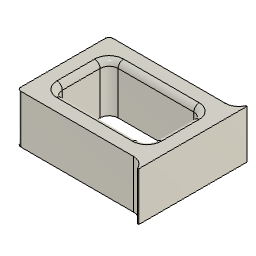
V0.2 Formbot Umbilical Panel Thermistor & 4-way Fan Bus v7 (Autodesk Fusion 360 design; units mm, degrees)
Autodesk Fusion 360 part; units mm, degrees
sketch "Fan Connector box" plane through (0, 0, 0) normal (0, 0, 1) x (1, 0, 0)
  line L0 (0, 0) -> (28.97, 0)
  line L1 (28.97, 0) -> (28.97, 7.7)
  line L2 (28.97, 7.7) -> (0, 7.7)
  line L3 (0, 7.7) -> (0, 0)
  dimension "d1" = 28.97
  dimension "d2" = 7.7
  constraint horizontal L0
  constraint vertical L1
  constraint horizontal L2
  constraint vertical L3
  constraint coincident L0.start L3.end
  measures "d1" distance of L0.start L0.end
  measures "d2" distance of L0.start L2.end
extrude "Extrude1" add sketch "Fan Connector box" along normal blind 6.5 makes body 1
shell "Shell1" thickness 1.2 outward yes removed faces 1 at (9.6567, 5.1333, 6.5) on bodies 1
chamfer "Chamfer1" distance 0.4 angle 45 4 edges at (14.485, 7.7, 6.5) (0, 3.85, 6.5) (14.485, 0, 6.5) (28.97, 3.85, 6.5) on bodies 1
sketch "v0.2 Formnot Umbilical Thermister Shroud" plane through (0, 0, 0) normal (0, 0, 1) x (1, 0, 0)
  line L0 (0, 23) -> (14.4, 23)
  line L1 (14.4, 23) -> (14.4, 12.8)
  line L2 (14.4, 12.8) -> (0, 12.8)
  line L3 (0, 12.8) -> (0, 23)
  circle A0 centre (12.9, 24.5) radius 1.5
  circle A1 centre (12.9, 11.3) radius 1.5
  line L4 (14.4, 12.8) -> (14.4, 11.3)
  line L5 (14.4, 23) -> (14.4, 24.5)
  dimension "d15" = 14.4
  dimension "d16" = 10.2
  dimension "d17" = 3
  dimension "d18" = 3
  constraint horizontal L0
  constraint vertical L1
  constraint horizontal L2
  constraint vertical L3
  constraint tangent L0 A0
  constraint tangent L1 A0
  constraint tangent L2 A1
  constraint tangent L1 A1
  constraint coincident A1 L4.end
  constraint tangent A1 L4
  constraint coincident A0 L5.end
  constraint tangent A0 L5
  measures "d15" distance of L0.start L0.end
  measures "d16" distance of L0.start L2.end
  measures "d17" diameter of A0
  measures "d18" diameter of A1
extrude "Extrude3" add sketch "v0.2 Formnot Umbilical Thermister Shroud" along normal blind 5.36 separate body contours L0 L1 L2 L3 | L0 A0 L5 | L2 A1 L4 makes body 2
shell "Shell2" thickness 2 removed faces 1 at (8.6, 19.6, 5.36) on bodies 2
extrude "Extrude4" cut 1 faces at (5.4667, 18.9333, 2) along direction (0, 0, -1) blind 2 on bodies 2 bodies 2
chamfer "Chamfer5" distance 0.6 angle 45 2 edges at (14.4, 24.5, 2.68) (14.4, 11.3, 2.68) on bodies 2
fillet "Fillet4" radius 0.4 2 edges at (0, 23, 2.68) (0, 12.8, 2.68) on bodies 2
fillet "Fillet5" radius 1 4 edges at (12.4, 21, 2.68) (2, 21, 2.68) (2, 14.8, 2.68) (12.4, 14.8, 2.68) on bodies 2
fillet "Fillet6" radius 0.6 8 edges at (12.1071, 20.7071, 5.36) (12.4, 17.9, 5.36) (12.1071, 15.0929, 5.36) (7.2, 14.8, 5.36) (2.2929, 15.0929, 5.36) (2, 17.9, 5.36) (2.2929, 20.7071, 5.36) (7.2, 21, 5.36) on bodies 2
hidden bodies 1
equation "d1 = ID_Length"
equation "d2 = ID_Width"
equation "ID_Width = 7.7 mm"
equation "ID_Length = 28.97 mm"
equation "ID_Height = 7.2 mm"
named bodies: "4-way Fan Connector box", "v0.2 Formbot Umbilical Thermister Shroud"
